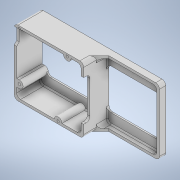
# Autodesk Inventor part: base
Saved by Autodesk Inventor 2021 (Build 250183000, 183)
## iProperties
Created: 2023-10-22
Part Number: base
Material: Generic
Document SubType Name: Modeling
Designer: Toby
Density: 1 g/cm^3
Appearance: Default
Author: Toby
Autodesk Inventor part; units mm, degrees
ref_plane "YZ Plane" through (0, 0, 0) normal (1, 0, 0) x (0, 1, 0)
ref_plane "XZ Plane" through (0, 0, 0) normal (0, 1, 0) x (-1, 0, 0)
ref_plane "XY Plane" through (0, 0, 0) normal (0, 0, 1) x (1, 0, 0)
sketch "Sketch1" plane through (0, 0, 0) normal (0, 0, 1) x (1, 0, 0)
  line L0 (-45.2903, 23.0196) -> (54.7097, 23.0196)
  line L1 (54.7097, 23.0196) -> (54.7097, -28.9804)
  line L2 (54.7097, -28.9804) -> (-45.2903, -28.9804)
  line L3 (-45.2903, -28.9804) -> (-45.2903, 23.0196)
  line L4 (-43.2903, 21.0196) -> (52.4644, 21.0196)
  line L5 (52.4644, 21.0196) -> (52.4644, -26.9804)
  line L6 (52.4644, -26.9804) -> (-43.2903, -26.9804)
  line L7 (-43.2903, -26.9804) -> (-43.2903, 21.0196)
  point P0 (0, 0)
  dimension "d0" = 100
  dimension "d1" = 52
  dimension "d2" = 2
  dimension "d3" = 2
  dimension "d4" = 2
  dimension "d5" = 2.2453
  constraints: 16 end point, 4 parallel, 2 horizontal, 2 perpendicular
  measures "d0" distance of L0.start L0.end
  measures "d1" distance of L2.end L0.start
  measures "d2" distance between parallel lines of L4 L0
  measures "d3" distance between parallel lines of L2 L6
  measures "d4" distance between parallel lines of L3 L7
  measures "d5" distance between parallel lines of L5 L1
extrude "Extrusion1" add sketch "Sketch1" along normal blind 20
sketch "Sketch2" plane through (0, 0, 20) normal (0, 0, 1) x (1, 0, 0)
  line L0 (-45.2903, 23.0196) -> (-45.2903, -28.9804) projected
  line L1 (-45.2903, -28.9804) -> (54.7097, -28.9804) projected
  circle A0 centre (-41.2903, 21.0196) radius 2
  circle A1 centre (-3.2903, 21.0196) radius 2
  circle A2 centre (-41.2903, -16.9804) radius 3
  circle A3 centre (-10.4903, -26.9804) radius 2
  line L2 (-43.2903, -26.9804) -> (-43.2903, 21.0196) projected
  line L3 (-41.2903, 21.0196) -> (-43.2903, 21.0196)
  line L4 (-43.2903, 21.0196) -> (-43.2903, 19.0196)
  line L5 (-43.2903, 19.0196) -> (-41.2903, 19.0196)
  line L6 (-41.2903, 19.0196) -> (-41.2903, 21.0196)
  line L7 (-41.2903, -13.9804) -> (-43.2903, -13.9804)
  line L8 (-43.2903, -13.9804) -> (-43.2903, -19.9804)
  line L9 (-43.2903, -19.9804) -> (-41.2903, -19.9804)
  line L10 (-41.2903, -19.9804) -> (-41.2903, -13.9804)
  point P0 (0, 0)
  dimension "d16" = 4
  dimension "d18" = 6
  dimension "d8" = 4
  dimension "d9" = 12
  dimension "d10" = 34.8
  dimension "d11" = 2
  dimension "d12" = 4
  dimension "d13" = 50
  dimension "d14" = 42
  dimension "d15" = 50
  dimension "d17" = 4
  dimension "d19" = 4
  dimension "d20" = 2
  constraints: 16 end point, 4 coincident, 4 parallel, 2 centre point, 2 horizontal, 2 perpendicular, 2 point on line, 5 other
  measures "d8" distance from line of L0 point (-41.29, -16.98)
  measures "d9" distance from line of L1 point (-41.29, -16.98)
  measures "d10" distance from line of L0 point (-10.49, -26.98)
  measures "d11" distance from line of L1 point (-10.49, -26.98)
  measures "d12" distance from line of L0 point (-41.29, 21.02)
  measures "d13" distance from line of L1 point (-41.29, 21.02)
  measures "d14" distance from line of L0 point (-3.29, 21.02)
  measures "d15" distance from line of L1 point (-3.29, 21.02)
  measures "d17" diameter of A1
  measures "d19" diameter of A3
  measures "d20" distance between parallel lines of L3 L5
extrude "Extrusion2" add sketch "Sketch2" against normal blind 20 contours A0 L6 L3 | L3 L6 A0 | A0 L5 L2 | A1 | A2 L10 | L10 A2 L2 | A2 L2 L7 | L9 L2 A2 | A3
sketch "Sketch3" plane through (0, 0, 20) normal (0, 0, 1) x (1, 0, 0)
  arc A0 (-41.2903, 19.0196) -> (-39.2903, 21.0196) centre (-41.2903, 21.0196) ccw projected
  arc A1 (-5.2903, 21.0196) -> (-1.2903, 21.0196) centre (-3.2903, 21.0196) ccw projected
  arc A2 (-41.2903, -19.9804) -> (-41.2903, -13.9804) centre (-41.2903, -16.9804) ccw projected
  arc A3 (-8.4903, -26.9804) -> (-12.4903, -26.9804) centre (-10.4903, -26.9804) ccw projected
  point P0 (0, 0)
  constraints: 4 coincident
hole "Hole1" at (-41.2903, 21.0196, 20) at (-3.2903, 21.0196, 20) at (-41.2903, -16.9804, 20) at (-10.4903, -26.9804, 20) direction (0, 0, -1) diameter 2 depth 10 tip angle 118
sketch "Sketch4" plane through (0, 0, 20) normal (0, 0, 1) x (1, 0, 0)
  line L0 (-1.2903, 21.0196) -> (52.4644, 21.0196) projected
  line L1 (52.4644, -26.9804) -> (-8.4903, -26.9804) projected
  line L2 (7.7097, 21.0196) -> (9.7097, 21.0196)
  line L3 (9.7097, 21.0196) -> (9.7097, -26.9804)
  line L4 (9.7097, -26.9804) -> (7.7097, -26.9804)
  line L5 (7.7097, -26.9804) -> (7.7097, 21.0196)
  line L6 (-45.2903, 23.0196) -> (-45.2903, -28.9804) projected
  point P0 (0, 0)
  dimension "d30" = 2
  dimension "d31" = 55
  constraints: 8 end point, 2 parallel, 2 point on line, 1 horizontal, 1 perpendicular
  measures "d30" distance between parallel lines of L3 L5
  measures "d31" distance between parallel lines of L6 L3
extrude "Extrusion3" add sketch "Sketch4" against normal blind 20
sketch "Sketch5" plane through (-45.2903, -28.9804, 0) normal (0, -1, 0) x (1, 0, 0)
  line L0 (100, 0) -> (100, 20) projected
  line L1 (55, 20) -> (55, 0) projected
  line L2 (100, 20) -> (55, 20)
  line L3 (55, 20) -> (55, 0)
  line L4 (55, 0) -> (100, 0)
  line L5 (100, 0) -> (100, 20)
  point P0 (45.2903, 0)
  constraints: 8 end point, 2 parallel, 1 horizontal, 1 perpendicular
extrude "Extrusion4" cut sketch "Sketch5" against normal blind 55
sketch "Sketch6" plane through (9.7097, -28.9804, 20) normal (1, 0, 0) x (0, 0, -1)
  line L0 (0, 2) -> (20, 2) projected
  line L1 (20, 0) -> (0, 0) projected
  line L2 (20, 2) -> (15, 2)
  line L3 (15, 2) -> (15, 0)
  line L4 (15, 0) -> (20, 0)
  line L5 (20, 0) -> (20, 2)
  line L6 (20, 52) -> (0, 52) projected
  line L7 (0, 50) -> (20, 50) projected
  line L8 (20, 52) -> (15, 52)
  line L9 (15, 52) -> (15, 50)
  line L10 (15, 50) -> (20, 50)
  line L11 (20, 50) -> (20, 52)
  point P0 (20, 28.9804)
  point P1 (15, 2)
  dimension "d36" = 5
  constraints: 16 end point, 4 parallel, 3 point on line, 2 horizontal, 2 perpendicular
  measures "d36" distance between parallel lines of L5 L3
extrude "Extrusion5" add sketch "Sketch6" along normal blind 5
chamfer "Chamfer1" distance 5 angle 45 2 edges at (9.7097, -27.9804, 5) (9.7097, 22.0196, 5)
fillet "Fillet1" radius 3 7 edges at (-43.2903, -26.9804, 10) (-45.2903, -28.9804, 10) (-45.2903, 23.0196, 10) (7.7097, 21.0196, 10) (9.7097, 23.0196, 15) (7.7097, -26.9804, 10) (9.7097, -28.9804, 15)
fillet "Fillet2" radius 3 5 edges at (9.5381, 21.0196, 5.0857) (4.7097, 21.0196, 10) (9.5381, -26.9804, 5.0857) (-40.2903, -26.9804, 10) (4.7097, -26.9804, 10)
sketch "Sketch7" plane through (9.7097, -25.9804, 20) normal (1, 0, 0) x (0, 0, -1)
  line L0 (0, 12) -> (0, 45) projected
  line L1 (0, -3) -> (7, -3) projected
  line L2 (0, 7) -> (5, 7)
  line L3 (5, 7) -> (5, 39)
  line L4 (5, 39) -> (0, 39)
  line L5 (0, 39) -> (0, 7)
  line L6 (7, 49) -> (0, 49) projected
  point P0 (20, 25.9804)
  point P1 (0, 23)
  point P2 (0, 39)
  point P3 (0, 12)
  dimension "d44" = 26
  dimension "d45" = 10
  dimension "d46" = 10
  dimension "d47" = 5
  constraints: 8 end point, 2 parallel, 2 point on line, 1 horizontal, 1 perpendicular
  measures "d44" distance from line of L1 point (0, 23)
  measures "d45" distance between parallel lines of L1 L2
  measures "d46" distance between parallel lines of L6 L4
  measures "d47" distance between parallel lines of L3 L0
extrude "Extrusion6" cut sketch "Sketch7" against normal blind 5
fillet "Fillet3" radius 3 2 edges at (8.7097, -18.9804, 15) (8.7097, 13.0196, 15)
sketch "Sketch8" plane through (0, 0, 20) normal (0, 0, 1) x (1, 0, 0)
  line L0 (-45.2903, 20.0196) -> (-45.2903, -25.9804) projected
  line L1 (-45.2903, 19.8196) -> (-37.0903, 19.8196)
  line L2 (-37.0903, 19.8196) -> (-37.0903, 9.0196)
  line L3 (-37.0903, 9.0196) -> (-45.2903, 9.0196)
  line L4 (-45.2903, 9.0196) -> (-45.2903, 19.8196)
  line L5 (6.7097, 23.0196) -> (-42.2903, 23.0196) projected
  point P0 (0, 0)
  dimension "d51" = 3.2
  dimension "d52" = 14
  dimension "d53" = 8.2
  constraints: 8 end point, 2 parallel, 1 horizontal, 1 perpendicular, 1 point on line
  measures "d51" distance between parallel lines of L1 L5
  measures "d52" distance between parallel lines of L3 L5
  measures "d53" distance between parallel lines of L0 L2
extrude "Extrusion7" cut sketch "Sketch8" against normal blind 2
chamfer "Chamfer2" distance 1 angle 45 2 edges at (-44.2903, 9.0196, 20) (-42.4903, 19.8196, 20)
chamfer "Chamfer3" distance 1 angle 45 2 edges at (-42.4903, 19.8196, 18) (-44.2903, 9.0196, 18)
sketch "Sketch9" plane through (0, 0, 0) normal (0, 0, -1) x (-1, 0, 0)
  line L0 (42.2903, -28.9804) -> (-14.7097, -28.9804) projected
  line L1 (-14.7097, -28.9804) -> (-54.7097, -28.9804)
  line L2 (-54.7097, -28.9804) -> (-54.7097, -26.9804)
  line L3 (-54.7097, -26.9804) -> (-14.7097, -26.9804)
  line L4 (-14.7097, -26.9804) -> (-14.7097, -28.9804)
  line L5 (-14.7097, 23.0196) -> (-14.7097, 21.0196) projected
  line L6 (-14.7097, 23.0196) -> (-54.7097, 23.0196)
  line L7 (-54.7097, 23.0196) -> (-54.7097, 21.0196)
  line L8 (-54.7097, 21.0196) -> (-14.7097, 21.0196)
  line L9 (-14.7097, 21.0196) -> (-14.7097, 23.0196)
  line L10 (-54.7097, -26.9804) -> (-52.7097, -26.9804)
  line L11 (-52.7097, -26.9804) -> (-52.7097, 21.0196)
  line L12 (-52.7097, 21.0196) -> (-54.7097, 21.0196)
  line L13 (-54.7097, 21.0196) -> (-54.7097, -26.9804)
  line L14 (45.2903, 20.0196) -> (45.2903, -25.9804) projected
  point P0 (0, 0)
  point P1 (-52.7097, -26.9804)
  point P2 (-52.7097, -26.9804)
  dimension "d62" = 2
  dimension "d63" = 100
  dimension "d64" = 2
  dimension "d65" = 2
  constraints: 24 end point, 6 parallel, 3 horizontal, 3 perpendicular, 1 collinear, 1 point on line
  measures "d62" distance between parallel lines of L11 L13
  measures "d63" distance between parallel lines of L14 L13
  measures "d64" distance between parallel lines of L1 L3
  measures "d65" distance between parallel lines of L6 L8
extrude "Extrusion8" add sketch "Sketch9" against normal blind 5
fillet "Fillet4" radius 3 4 edges at (52.7097, -26.9804, 2.5) (54.7097, -28.9804, 2.5) (52.7097, 21.0196, 2.5) (54.7097, 23.0196, 2.5)
sketch "Sketch10" plane through (0, 0, 20) normal (0, 0, 1) x (1, 0, 0)
  circle A0 centre (-3.2903, 21.0196) radius 1 projected
  circle A1 centre (-3.2903, 21.0196) radius 3
  circle A2 centre (-3.2903, 21.0196) radius 2
  line L0 (-39.2903, 21.0196) -> (-5.2903, 21.0196) projected
  arc A3 (-5.2903, 21.0196) -> (-1.2903, 21.0196) centre (-3.2903, 21.0196) ccw projected
  line L1 (-6.2903, 21.0196) -> (-5.2903, 21.0196)
  line L2 (-5.2903, 21.0196) -> (-1.2903, 21.0196)
  line L3 (-1.2903, 21.0196) -> (4.7097, 21.0196) projected
  line L4 (-0.1876, 21.0196) -> (-1.2903, 21.0196)
  point P0 (0, 0)
  point P1 (-0.2903, 21.0196)
  dimension "d69" = 6
  constraints: 6 end point, 2 coincident, 2 point on line, 1 centre point, 1 collinear, 1 horizontal, 1 point on circle, 3 other
extrude "Extrusion9" add sketch "Sketch10" against normal blind 20 contours L3 A1 L0 A2 picked at (-0.6721, 20.6207)
sketch "Sketch11" plane through (0, 0, 20) normal (0, 0, 1) x (1, 0, 0)
  circle A0 centre (-10.4903, -26.9804) radius 1 projected
  circle A1 centre (-10.4903, -26.9804) radius 3
  circle A2 centre (-10.4903, -26.9804) radius 2
  line L0 (-12.4903, -26.9804) -> (-40.2903, -26.9804) projected
  line L1 (-13.4903, -26.9804) -> (-7.4903, -26.9804)
  point P0 (0, 0)
  point P1 (-8.4903, -26.9804)
  dimension "d73" = 4
  dimension "d72" = 6
  constraints: 2 coincident, 2 end point, 2 point on circle, 1 centre point, 1 collinear, 1 point on line, 2 other
  measures "d72" diameter of A1
extrude "Extrusion10" add sketch "Sketch11" against normal blind 20 contours A2 L0 A1 L1 picked at (-8.795, -24.9456)
sketch "Sketch12" plane through (0, 0, 0) normal (0, 0, -1) x (-1, 0, 0)
  line L0 (43.2903, -26.9804) -> (-52.7097, -26.9804)
  line L1 (-52.7097, -26.9804) -> (-52.7097, -18.9804)
  line L2 (-52.7097, -18.9804) -> (43.2903, -18.9804)
  line L3 (43.2903, -18.9804) -> (43.2903, -26.9804)
  line L4 (-52.7097, -23.9804) -> (-52.7097, 18.0196) projected
  line L5 (43.2903, 21.0196) -> (-52.7097, 21.0196)
  line L6 (-52.7097, 21.0196) -> (-52.7097, 13.0196)
  line L7 (-52.7097, 13.0196) -> (43.2903, 13.0196)
  line L8 (43.2903, 13.0196) -> (43.2903, 21.0196)
  line L9 (43.2903, -13.9804) -> (43.2903, 19.0196) projected
  line L10 (39.2903, 21.0196) -> (6.2903, 21.0196) projected
  line L11 (-12.7097, -26.9804) -> (-49.7097, -26.9804) projected
  line L12 (43.2903, -23.9804) -> (43.2903, -19.9804) projected
  line L13 (42.2903, -28.9804) -> (-51.7097, -28.9804) projected
  line L14 (-51.7097, 23.0196) -> (42.2903, 23.0196) projected
  point P0 (0, 0)
  dimension "d76" = 10
  dimension "d77" = 10
  constraints: 16 end point, 5 collinear, 4 parallel, 2 horizontal, 2 perpendicular, 1 point on line
  measures "d76" distance between parallel lines of L2 L13
  measures "d77" distance between parallel lines of L14 L7
extrude "Extrusion11" add sketch "Sketch12" against normal blind 1.2
fillet "Fillet5" radius 3 4 edges at (-39.0543, -18.9804, 0.6) (52.7097, -18.9804, 0.6) (52.7097, 13.0196, 0.6) (-43.2903, 13.0196, 0.6)
fillet "Fillet6" radius 3 4 edges at (7.7097, -18.9804, 0.6) (9.7097, -18.9804, 0.6) (7.7097, 13.0196, 0.6) (9.7097, 13.0196, 0.6)
chamfer "Chamfer4" distance 1 angle 45 10 edges at (9.7097, 15.5196, 1.2) (9.7097, -21.4804, 1.2) (10.5884, -26.1018, 1.2) (31.2097, -26.9804, 1.2) (51.831, -26.1018, 1.2) (52.7097, -21.4804, 1.2) (10.5884, 20.1409, 1.2) (31.2097, 21.0196, 1.2) (51.831, 20.1409, 1.2) (52.7097, 15.5196, 1.2)
chamfer "Chamfer5" distance 1 angle 45 11 edges at (-26.8903, -26.9804, 1.2) (-1.3903, -26.9804, 1.2) (-42.4116, -26.1018, 1.2) (-43.2903, -21.9804, 1.2) (6.831, -26.1018, 1.2) (7.7097, 15.5196, 1.2) (7.7097, -21.4804, 1.2) (-22.7903, 21.0196, 1.2) (-43.2903, 16.0196, 1.2) (6.831, 20.1409, 1.2) (2.2097, 21.0196, 1.2)
body "Solid1"
